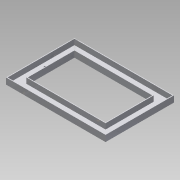
# Autodesk Inventor part: Catch pan
Saved by Autodesk Inventor 2015 (Build 190159000, 159)
## iProperties
Created: 2015-05-27
Part Number: Catch pan
Material: Aluminum 6061
Document SubType Name: Modeling
Designer: Joe Sheldon
Density: 2.7 g/cm^3
Appearance: Aluminum - Flat
Author: Joe Sheldon
Autodesk Inventor part; units mm, degrees
ref_plane "YZ Plane" through (0, 0, 0) normal (1, 0, 0) x (0, 1, 0)
ref_plane "XZ Plane" through (0, 0, 0) normal (0, 1, 0) x (-1, 0, 0)
ref_plane "XY Plane" through (0, 0, 0) normal (0, 0, 1) x (1, 0, 0)
sketch "Sketch3" plane through (0, 0, 0) normal (0, 1, 0) x (-1, 0, 0)
  line L0 (-203.2, 139.7) -> (203.2, 139.7)
  line L1 (203.2, 139.7) -> (203.2, -139.7)
  line L2 (203.2, -139.7) -> (-203.2, -139.7)
  line L3 (-203.2, -139.7) -> (-203.2, 139.7)
  line L4 (-203.2, 139.7) -> (203.2, -139.7) construction
  line L5 (203.2, 139.7) -> (-203.2, -139.7) construction
  line L6 (152.4, -88.9) -> (152.4, 88.9)
  line L7 (152.4, 88.9) -> (-152.4, 88.9)
  line L8 (-152.4, 88.9) -> (-152.4, -88.9)
  line L9 (-152.4, -88.9) -> (152.4, -88.9)
  line L10 (158.75, -95.25) -> (158.75, 95.25)
  line L11 (158.75, 95.25) -> (-158.75, 95.25)
  line L12 (-158.75, 95.25) -> (-158.75, -95.25)
  line L13 (-158.75, -95.25) -> (158.75, -95.25)
  point P0 (0, 0)
  dimension "d11" = 406.4
  dimension "d12" = 279.4
  dimension "d13" = 50.8
  dimension "d14" = 44.45
  constraints: 28 end point, 6 parallel, 3 perpendicular, 2 midpoint, 1 horizontal, 6 other
  measures "d11" distance of L1.end L2.end
  measures "d12" distance of L0.end L1.end
  measures "d13" distance between parallel lines of L1 L6
  measures "d14" distance between parallel lines of L1 L10
extrude "Extrusion3" add sketch "Sketch3" along normal blind 50.8 contours L0 L1 L2 L3
shell "Shell2" thickness 3.175 removed faces 1 at (52.9167, 50.8, -124.8833)
sketch "Sketch4" plane through (0, 50.8, 0) normal (0, 1, 0) x (1, 0, 0)
  line L0 (227.9599, -165.6341) -> (-227.9599, -165.6341)
  line L1 (-227.9599, -165.6341) -> (-227.9599, 165.6341)
  line L2 (-227.9599, 165.6341) -> (227.9599, 165.6341)
  line L3 (227.9599, 165.6341) -> (227.9599, -165.6341)
  line L4 (227.9599, -165.6341) -> (-227.9599, 165.6341) construction
  line L5 (-227.9599, -165.6341) -> (227.9599, 165.6341) construction
  point P0 (0, 0)
  constraints: 12 end point, 2 midpoint, 2 parallel, 1 horizontal, 1 perpendicular
extrude "Extrusion4" cut sketch "Sketch4" against normal blind 25.4
sketch "Sketch5" plane through (-200.025, 3.175, 136.525) normal (0, 1, 0) x (1, 0, 0)
  line L0 (361.95, 234.95) -> (38.1, 234.95) projected
  line L1 (361.95, 38.1) -> (361.95, 234.95) projected
  line L2 (38.1, 38.1) -> (361.95, 38.1) projected
  line L3 (38.1, 234.95) -> (38.1, 38.1) projected
  line L4 (400.05, 0) -> (0, 0) projected
  line L5 (400.05, 273.05) -> (400.05, 0) projected
  line L6 (0, 273.05) -> (400.05, 273.05) projected
  line L7 (0, 0) -> (0, 273.05) projected
  line L8 (38.1, 38.1) -> (0, 38.1)
  line L9 (0, 38.1) -> (0, 234.95)
  line L10 (0, 234.95) -> (38.1, 234.95)
  line L11 (38.1, 234.95) -> (38.1, 38.1)
  circle A0 centre (19.05, 136.525) radius 6.35
  point P0 (200.025, 136.525)
  dimension "d20" = 12.7
  constraints: 8 end point, 2 parallel, 1 centre point, 1 horizontal, 1 perpendicular, 1 point on line
  measures "d20" diameter of A0
extrude "Extrusion5" cut sketch "Sketch5" against normal blind 25.4 contours A0
body "Solid3"
